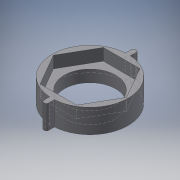
# Autodesk Inventor part: tensioner
Saved by Autodesk Inventor 2017 (Build 210142000, 142)
## iProperties
Created: 2017-06-23
Part Number: tensioner
Material: Generic
Document SubType Name: Modeling
Designer: erwin
Density: 1 g/cm^3
Appearance: Default
Author: erwin
Autodesk Inventor part; units mm, degrees
ref_plane "YZ Plane" through (0, 0, 0) normal (1, 0, 0) x (0, 1, 0)
ref_plane "XZ Plane" through (0, 0, 0) normal (0, 1, 0) x (-1, 0, 0)
ref_plane "XY Plane" through (0, 0, 0) normal (0, 0, 1) x (1, 0, 0)
sketch "Sketch1" plane through (0, 0, 0) normal (0, 0, 1) x (1, 0, 0)
  arc A0 (-2.9865, -4.9749) -> (-2.9865, 4.9749) centre (-3.4865, 0) ccw
  arc A1 (-3.9865, 4.9749) -> (-3.9865, -4.9749) centre (-3.4865, 0) ccw
  line L0 (-3.9865, 4.9749) -> (-3.9865, 5.9791)
  arc A2 (-2.9865, 5.9791) -> (-3.9865, 5.9791) centre (-3.4865, 0) ccw
  line L1 (-2.9865, 5.9791) -> (-2.9865, 4.9749)
  line L2 (-3.9865, -5.9791) -> (-3.9865, -4.9749)
  arc A3 (-3.9865, -5.9791) -> (-2.9865, -5.9791) centre (-3.4865, 0) ccw
  line L3 (-2.9865, -4.9749) -> (-2.9865, -5.9791)
  arc A4 (-3.7865, 4.7906) -> (-3.7865, -4.7906) centre (-3.4865, 0) ccw
  line L4 (-3.7865, 4.7906) -> (-3.7865, 5.5498)
  arc A5 (-3.4343, 5.7998) -> (-3.5388, 5.7998) centre (-3.4865, 0) ccw
  line L5 (-3.1865, 5.5498) -> (-3.1865, 4.7906)
  arc A6 (-3.1865, -4.7906) -> (-3.1865, 4.7906) centre (-3.4865, 0) ccw
  line L6 (-3.1865, -4.7906) -> (-3.1865, -5.5498)
  arc A7 (-3.5388, -5.7998) -> (-3.4343, -5.7998) centre (-3.4865, 0) ccw
  line L7 (-3.7865, -5.5498) -> (-3.7865, -4.7906)
  arc A8 (-3.5388, 5.7998) -> (-3.7865, 5.5498) centre (-3.5365, 5.5498) ccw
  arc A9 (-3.1865, 5.5498) -> (-3.4343, 5.7998) centre (-3.4365, 5.5498) ccw
  arc A10 (-3.4343, -5.7998) -> (-3.1865, -5.5498) centre (-3.4365, -5.5498) ccw
  arc A11 (-3.7865, -5.5498) -> (-3.5388, -5.7998) centre (-3.5365, -5.5498) ccw
  point P0 (0, 0)
  point P1 (-3.7865, 5.7922)
  point P2 (-3.1865, 5.7922)
  point P3 (-3.1865, -5.7922)
  point P4 (-3.7865, -5.7922)
  dimension "d2" = 0.2
  dimension "d3" = 0.25
  constraints: 28 point on circle, 16 end point, 12 centre point, 8 tangent, 4 point on line, 3 equal radius, 7 other
  measures "d2" radial gap between concentric circles of A1 A4
  measures "d3" radius of A8
extrude "Extrusion1" add sketch "Sketch1" along normal blind 3 contours L4 A8 A5 A9 L5 A6 L6 A10 A7 A11 L7 A4
sketch "Sketch2" plane through (0, 0, 3) normal (0, 0, 1) x (1, 0, 0)
  circle A0 centre (-3.4865, 0) radius 1.5 projected
  line L0 (-1.1771, -4) -> (-5.7959, -4)
  line L1 (-5.7959, -4) -> (-8.1053, 0)
  line L2 (-8.1053, 0) -> (-5.7959, 4)
  line L3 (-5.7959, 4) -> (-1.1771, 4)
  line L4 (-1.1771, 4) -> (1.1323, 0)
  line L5 (1.1323, 0) -> (-1.1771, -4)
  point P0 (0, 0)
  dimension "d6" = 8
  constraints: 12 end point, 1 coincident, 13 other
  measures "d6" distance between parallel lines of L2 L5
extrude "Extrusion2" cut sketch "Sketch2" against normal blind 1
hole "Hole1" at (-3.4865, 0, 3) direction (0, 0, -1) diameter 6.5 depth 8 tip angle 118
move faces "Move1" translate (0, 0, -0.5) faces at (-6.6875, 1.9487, 2)
body "Solid1"
